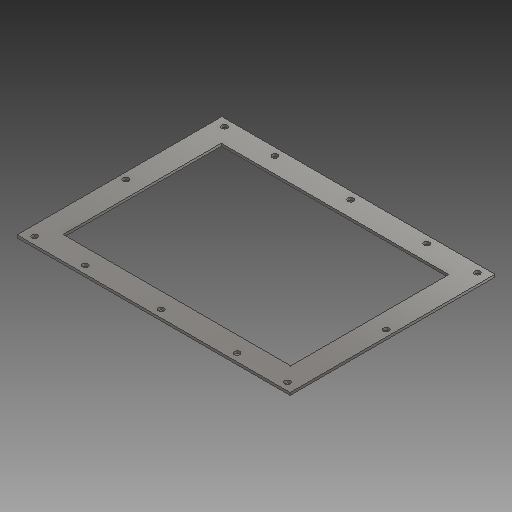
# Autodesk Inventor part: Gegenhalter
Saved by Autodesk Inventor 2018 (Build 220112000, 112)
## iProperties
Created: 2017-10-08
Part Number: Gegenhalter
Material: Edelstahl
Document SubType Name: Blech
Designer: jro
Density: 8 g/cm^3
Sheet Metal Rule: Standard_mm
Appearance: Halbpoliert
Author: jro
Autodesk Inventor part; units mm, degrees
ref_plane "YZ Plane" through (0, 0, 0) normal (1, 0, 0) x (0, 1, 0)
ref_plane "XZ Plane" through (0, 0, 0) normal (0, 1, 0) x (-1, 0, 0)
ref_plane "XY Plane" through (0, 0, 0) normal (0, 0, 1) x (1, 0, 0)
sketch "Skizze1" plane through (0, 0, 0) normal (0, 0, 1) x (1, 0, 0)
  line L0 (-108, 81) -> (-108, -81)
  line L1 (108, 81) -> (-108, 81)
  line L2 (-108, -81) -> (108, -81)
  line L3 (108, -81) -> (108, 81)
  line L4 (-90, 62.5) -> (90, 62.5)
  line L5 (90, 62.5) -> (90, -62.5)
  line L6 (90, -62.5) -> (-90, -62.5)
  line L7 (-90, -62.5) -> (-90, 62.5)
  circle A0 centre (100, -75) radius 2.25
  circle A1 centre (60, -75) radius 2.25
  circle A2 centre (0, -75) radius 2.25
  circle A3 centre (-60, -75) radius 2.25
  circle A4 centre (-100, -75) radius 2.25
  circle A5 centre (103, 0) radius 2.25
  circle A6 centre (-103, 0) radius 2.25
  circle A7 centre (100, 75) radius 2.25
  circle A8 centre (60, 75) radius 2.25
  circle A9 centre (0, 75) radius 2.25
  circle A10 centre (-60, 75) radius 2.25
  circle A11 centre (-100, 75) radius 2.25
  line L8 (-108, 81) -> (108, 81)
  line L9 (108, 81) -> (108, -81)
  line L10 (108, -81) -> (-108, -81)
  line L11 (-108, -81) -> (-108, 81)
  line L12 (90, 62.5) -> (-90, 62.5)
  line L13 (-90, 62.5) -> (-90, -62.5)
  line L14 (-90, -62.5) -> (90, -62.5)
  line L15 (90, -62.5) -> (90, 62.5)
  dimension "d1" = 180
  dimension "d2" = 125
  dimension "d3" = 162
  dimension "d4" = 216
  measures "d1" distance of L4.start L4.end
  measures "d2" distance of L5.start L5.end
  measures "d3" distance of L3.start L3.end
  measures "d4" distance of L1.start L1.end
extrude "Grobblech2" add sketch "Skizze1" along normal blind 2
equation "\"d5\" = Stärke"
equation "\"Biegeradius\" = Stärke"
equation "\"BreiteBiegungsfreistellung\" = Stärke"
equation "\"TiefeBiegungsfreistellung\" = 0.5 * Stärke"
equation "\"GrößeEckenfreistellung\" = 4 * Stärke"
equation "\"MinimalRest\" = 2 * Stärke"
equation "\"Übergangsradius\" = Biegeradius"
equation "\"JacobiRadiusGröße\" = Biegeradius"
equation "\"Abstandsgröße\" = Stärke"
equation "\"Stärke\" = 2"
